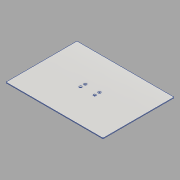
# Autodesk Inventor part: PBLMK-041-2
Saved by Autodesk Inventor 2016 (Build 200138000, 138)
## iProperties
Created: 2023-12-03
Part Number: PBLMK-041-2
Material: Aluminum
Document SubType Name: Modeling
Designer: Riskinova Oktavia
Density: 2.7 g/cm^3
Appearance: Aluminum - Flat
Description: BASE
Author: Riskinova Oktavia
Autodesk Inventor part; units mm, degrees
ref_plane "YZ Plane" through (0, 0, 0) normal (1, 0, 0) x (0, 1, 0)
ref_plane "XZ Plane" through (0, 0, 0) normal (0, 1, 0) x (-1, 0, 0)
ref_plane "XY Plane" through (0, 0, 0) normal (0, 0, 1) x (1, 0, 0)
sketch "Sketch1" plane through (0, 0, 0) normal (0, 0, 1) x (1, 0, 0)
  line L0 (-205, -150) -> (205, -150)
  line L1 (205, -150) -> (205, 150)
  line L2 (205, 150) -> (-205, 150)
  line L3 (-205, 150) -> (-205, -150)
  line L4 (-205, -150) -> (205, 150) construction
  line L5 (205, -150) -> (-205, 150) construction
  point P0 (0, 0)
  dimension "d0" = 410
  dimension "d1" = 300
  constraints: 12 end point, 2 midpoint, 2 parallel, 1 horizontal, 1 perpendicular
  measures "d0" distance of L1.end L2.end
  measures "d1" distance of L0.end L1.end
extrude "Extrusion1" add sketch "Sketch1" along normal mid plane 3
sketch "Sketch5" plane through (0, 0, 1.5) normal (0, 0, 1) x (1, 0, 0)
  circle A0 centre (-30, 10) radius 2.1 projected
  circle A1 centre (-30, -10) radius 2.1 projected
  circle A2 centre (30, 10) radius 2.1 projected
  circle A3 centre (30, -10) radius 2.1 projected
  point P0 (0, 0)
  constraints: 4 coincident
hole "Hole2" at (-30, 10, 1.5) at (-30, -10, 1.5) at (30, 10, 1.5) at (30, -10, 1.5) direction (0, 0, -1) diameter 5.5 end through all countersink diameter 11 countersink angle 90 clearance for "Countersunk Flat Head Screw ISO 2009/7046" size "M5" standard "ISO"
fillet "Fillet2" radius 3 4 edges at (205, -150, 0) (205, 150, 0) (-205, 150, 0) (-205, -150, 0)
body "Solid1"
